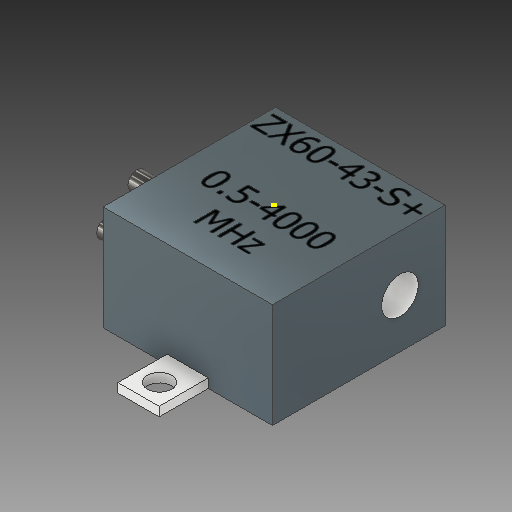
# Autodesk Inventor part: USB-1SP16T-83H-01
Saved by Autodesk Inventor 2018 (Build 220112000, 112)
## iProperties
Created: 2019-09-24
Part Number: USB-1SP16T-83H-01
Material: Generic
Document SubType Name: Modeling
Designer: alexanderpollak
Density: 1 g/cm^3
Appearance: Denim - Blue
Author: alexanderpollak
Autodesk Inventor part; units mm, degrees
ref_plane "YZ Plane" through (0, 0, 0) normal (1, 0, 0) x (0, 1, 0)
ref_plane "XZ Plane" through (0, 0, 0) normal (0, 1, 0) x (-1, 0, 0)
ref_plane "XY Plane" through (0, 0, 0) normal (0, 0, 1) x (1, 0, 0)
sketch "Sketch1" plane through (0, 0, 0) normal (0, 1, 0) x (-1, 0, 0)
  line L0 (9.4, 9.575) -> (-9.4, 9.575)
  line L1 (-9.4, 9.575) -> (-9.4, -9.575)
  line L2 (-9.4, -9.575) -> (9.4, -9.575)
  line L3 (9.4, -9.575) -> (9.4, 9.575)
  line L4 (9.4, 9.575) -> (-9.4, -9.575) construction
  line L5 (-9.4, 9.575) -> (9.4, -9.575) construction
  point P0 (0, 0)
  dimension "d0" = 18.8
  dimension "d1" = 19.15
  constraints: 12 end point, 2 midpoint, 2 parallel, 1 horizontal, 1 perpendicular
  measures "d0" distance of L2.end L1.end
  measures "d1" distance between parallel lines of L0 L2
extrude "Extrusion1" add sketch "Sketch1" along normal blind 11.61
sketch "Sketch6" plane through (9.4, 0, 9.575) normal (1, 0, 0) x (0, 0, -1)
  line L0 (0, 0) -> (19.15, 0) projected
  line L1 (0, 0) -> (0, 11.61) projected
  line L2 (19.15, 0) -> (19.15, 11.61) projected
  point P0 (9.575, 0)
  point P1 (14.15, 5.44)
  dimension "d60" = 5.44
  dimension "d76" = 5
  measures "d60" distance from line of point (14.15, 5.44) L0
  measures "d76" distance from line of L2 point (14.15, 5.44)
hole "Hole6" at (9.4, 5.44, -4.575) direction (-1, 0, 0) diameter 4.077 depth 5
sketch "Sketch7" plane through (-9.4, 0, -9.575) normal (-1, 0, 0) x (0, 0, 1)
  circle A0 centre (5, 5.44) radius 2.0385 projected
  point P0 (9.575, 0)
  constraints: 1 coincident
hole "Hole7" at (-9.4, 5.44, -4.575) direction (1, 0, 0) diameter 4.077 depth 5
sketch "Sketch8" plane through (0, 11.61, 0) normal (0, 1, 0) x (1, 0, 0)
  line L0 (-37.5313, 24.2217) -> (38.0409, 24.2217) construction
  line L1 (38.0409, 24.2217) -> (38.0409, -24.8493) construction
  line L2 (38.0409, -24.8493) -> (-37.5313, -24.8493) construction
  line L3 (-37.5313, -24.8493) -> (-37.5313, 24.2217) construction
  point P0 (0, 0)
  constraints: 2 other
sketch "Sketch9" plane through (0, 0, 0) normal (0, -1, 0) x (1, 0, 0)
  line L0 (2.285, 15.035) -> (-2.285, 15.035)
  line L1 (-2.285, 15.035) -> (-2.285, -15.035)
  line L2 (-2.285, -15.035) -> (2.285, -15.035)
  line L3 (2.285, -15.035) -> (2.285, 15.035)
  line L4 (2.285, 15.035) -> (-2.285, -15.035) construction
  line L5 (-2.285, 15.035) -> (2.285, -15.035) construction
  point P0 (0, 0)
  dimension "d77" = 4.57
  dimension "d78" = 30.07
  constraints: 12 end point, 2 midpoint, 2 parallel, 1 horizontal, 1 perpendicular
  measures "d77" distance of L2.end L1.end
  measures "d78" distance of L1.end L0.end
extrude "Extrusion2" add sketch "Sketch9" against normal blind 1.02
sketch "Sketch10" plane through (0, 0, 0) normal (0, -1, 0) x (1, 0, 0)
  line L0 (-2.285, -15.035) -> (2.285, -15.035) construction
  line L1 (0, -15.035) -> (0, 15.035) construction
  line L2 (-2.285, 15.035) -> (2.285, 15.035) construction
  point P0 (0, 0)
  point P1 (0, -12.7)
  point P2 (0, 12.7)
  dimension "d81" = 12.7
  dimension "d82" = 12.7
  constraints: 2 end point, 2 midpoint, 2 point on line
  measures "d81" distance of point (0, -12.7) point (0, 0)
  measures "d82" distance of point (0, 0) point (0, 12.7)
hole "Hole8" at (0, 0, -12.7) at (0, 0, 12.7) direction (0, 1, 0) diameter 2.7 end through all
sketch "Sketch11" plane through (-9.4, 0, -9.575) normal (-1, 0, 0) x (0, 0, 1)
  circle A0 centre (11.4, 8.31) radius 1
  circle A1 centre (14.86, 5.44) radius 1
  line L0 (0, 0) -> (19.15, 0) projected
  line L1 (0, 0) -> (0, 11.61) projected
  point P0 (9.575, 0)
  dimension "d90" = 2
  dimension "d91" = 2
  dimension "d92" = 5.44
  dimension "d93" = 8.31
  dimension "d94" = 14.86
  dimension "d95" = 11.4
  constraints: 2 centre point
  measures "d90" diameter of A0
  measures "d91" diameter of A1
  measures "d92" distance from line of A1.centre L0
  measures "d93" distance from line of A0.centre L0
  measures "d94" distance from line of A1.centre L1
  measures "d95" distance from line of A0.centre L1
extrude "Extrusion3" add sketch "Sketch11" along normal blind 4
sketch "Sketch12" plane through (0, 11.61, 0) normal (0, 1, 0) x (1, 0, 0)
  line L0 (-9.2157, 9.4666) -> (9.3495, 9.4666) construction
  line L1 (9.3495, 9.4666) -> (9.3495, -9.4331) construction
  line L2 (9.3495, -9.4331) -> (-9.2157, -9.4331) construction
  line L3 (-9.2157, -9.4331) -> (-9.2157, 9.4666) construction
  point P0 (0, 0)
  constraints: 2 other
body "Solid1"
